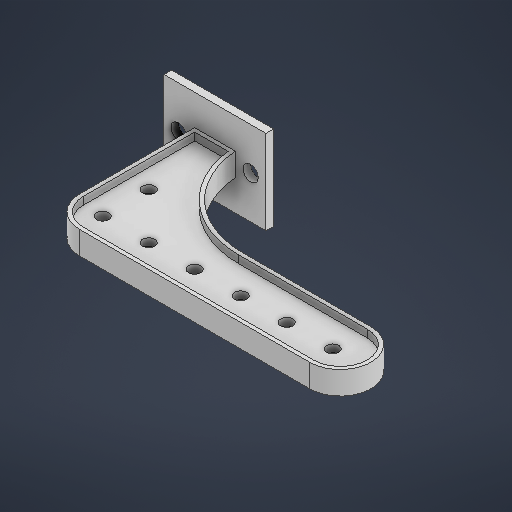
# Autodesk Inventor part: Pylon2
Saved by Autodesk Inventor 2026.1 (Build 301233000, 233)
## iProperties
Created: 2025-09-15
Part Number: Pylon2
Material: Generic
Document SubType Name: Modeling
Designer: mateo
Density: 1 g/cm^3
Appearance: Default
Author: mateo
Autodesk Inventor part; units mm, degrees
ref_plane "YZ Plane" through (0, 0, 0) normal (1, 0, 0) x (0, 1, 0)
ref_plane "XZ Plane" through (0, 0, 0) normal (0, 1, 0) x (-1, 0, 0)
ref_plane "XY Plane" through (0, 0, 0) normal (0, 0, 1) x (1, 0, 0)
sketch "Sketch1" plane through (0, 0, 0) normal (0, 1, 0) x (-1, 0, 0)
  line L0 (0, 0) -> (80, 0)
  line L1 (20, 5) -> (0, 5)
  line L2 (0, 5) -> (0, 0)
  line L3 (46.5184, 5) -> (46.5184, 80)
  circle A0 centre (26.5184, 80) radius 20
  line L4 (26.5184, 100) -> (-123.4816, 100)
  circle A1 centre (-123.4816, 80) radius 20
  line L5 (-123.4816, 60) -> (-39.7913, 60)
  arc A2 (20, 5) -> (-39.7913, 60) centre (-39.7913, 0) ccw
  line L6 (46.5184, 5) -> (66.5184, 5)
  line L7 (66.5184, 5) -> (66.5184, 0)
  line L8 (66.5184, 0) -> (46.5184, 0)
  point P0 (16.5184, 60)
  dimension "d1" = 75
  dimension "d2" = 40
  dimension "d3" = 150
  dimension "d4" = 140
  dimension "d7" = 40
  dimension "d10" = 5
  dimension "d11" = 5
  constraints: 18 end point, 6 point on circle, 4 horizontal, 3 centre point, 3 tangent, 2 parallel, 1 perpendicular, 1 point on line, 1 vertical
  measures "d1" distance of L3.start L3.end
  measures "d2" diameter of A0
  measures "d3" distance of L4.start L4.end
  measures "d4" distance of L5.start point (16.518, 60)
  measures "d7" diameter of A1
  measures "d10" distance of L6.end L7.end
  measures "d11" distance of L1.end L0.start
extrude "Extrusion1" add sketch "Sketch1" along normal blind 15
sketch "Sketch4" plane through (0, 0, 0) normal (0, -1, 0) x (1, 0, 0)
  line L0 (-26.5184, 100) -> (123.4816, 100) projected
  arc A0 (-26.5184, 100) -> (-46.5184, 80) centre (-26.5184, 80) ccw projected
  line L1 (-46.5184, 5) -> (-46.5184, 80) projected
  line L2 (-66.5184, 5) -> (-46.5184, 5) projected
  line L3 (-66.5184, 0) -> (-66.5184, 5) projected
  line L4 (0, 0) -> (-66.5184, 0) projected
  line L5 (0, 5) -> (0, 0) projected
  line L6 (-20, 5) -> (0, 5) projected
  arc A1 (39.7913, 60) -> (-20, 5) centre (39.7913, 0) ccw projected
  line L7 (123.4816, 60) -> (39.7913, 60) projected
  arc A2 (123.4816, 60) -> (123.4816, 100) centre (123.4816, 80) ccw projected
  line L8 (-20, 5) -> (-46.5184, 5)
  constraints: 2 end point, 1 horizontal
extrude "Extrusion3" add sketch "Sketch4" along normal blind 20 and the other way blind 35 contours L8 L6 L5 L4 L3 L2
sketch "Sketch5" plane through (0, 0, 0) normal (0, -1, 0) x (1, 0, 0)
  line L0 (-46.5184, 5) -> (-20, 5) projected
  arc A0 (39.7913, 60) -> (-20, 5) centre (39.7913, 0) ccw projected
  line L1 (123.4816, 60) -> (39.7913, 60) projected
  arc A1 (123.4816, 60) -> (123.4816, 100) centre (123.4816, 80) ccw projected
  line L2 (-26.5184, 100) -> (123.4816, 100) projected
  arc A2 (-26.5184, 100) -> (-46.5184, 80) centre (-26.5184, 80) ccw projected
  line L3 (-46.5184, 5) -> (-46.5184, 80) projected
  arc A3 (39.7913, 62.5) -> (-22.2571, 7.5) centre (39.7913, 0) ccw
  line L4 (-22.2571, 7.5) -> (-44.0184, 7.5)
  line L5 (-44.0184, 7.5) -> (-44.0184, 80)
  arc A4 (-26.5184, 97.5) -> (-44.0184, 80) centre (-26.5184, 80) ccw
  line L6 (-26.5184, 97.5) -> (123.4816, 97.5)
  arc A5 (123.4816, 62.5) -> (123.4816, 97.5) centre (123.4816, 80) ccw
  line L7 (123.4816, 62.5) -> (39.7913, 62.5)
  point P0 (0, 0)
  dimension "d29" = 2.5
  constraints: 8 end point, 6 point on circle, 3 centre point, 6 other
  measures "d29" distance between parallel lines of L1 L7
extrude "Extrusion4" cut sketch "Sketch5" against normal blind 5 contours A3 L4 L5 A4 L6 A5 L7
sketch "Sketch6" plane through (0, 15, 0) normal (0, 1, 0) x (1, 0, 0)
  line L0 (-20, -5) -> (-46.5184, -5) projected
  line L1 (-46.5184, -5) -> (-46.5184, -80) projected
  arc A0 (-46.5184, -80) -> (-26.5184, -100) centre (-26.5184, -80) ccw projected
  line L2 (-26.5184, -100) -> (123.4816, -100) projected
  arc A1 (123.4816, -100) -> (123.4816, -60) centre (123.4816, -80) ccw projected
  line L3 (123.4816, -60) -> (39.7913, -60) projected
  arc A2 (-20, -5) -> (39.7913, -60) centre (39.7913, 0) ccw projected
  line L4 (-44.0184, -80) -> (-44.0184, -7.5)
  line L5 (-44.0184, -7.5) -> (-22.2571, -7.5)
  arc A3 (-22.2571, -7.5) -> (39.7913, -62.5) centre (39.7913, 0) ccw
  line L6 (39.7913, -62.5) -> (123.4816, -62.5)
  arc A4 (123.4816, -97.5) -> (123.4816, -62.5) centre (123.4816, -80) ccw
  line L7 (123.4816, -97.5) -> (-26.5184, -97.5)
  arc A5 (-44.0184, -80) -> (-26.5184, -97.5) centre (-26.5184, -80) ccw
  point P0 (0, 0)
  dimension "d32" = 2.5
  constraints: 8 end point, 6 point on circle, 3 centre point, 6 other
  measures "d32" distance between parallel lines of L1 L4
extrude "Extrusion5" cut sketch "Sketch6" against normal blind 5 contours L4 L5 A3 L6 A4 L7 A5
sketch "Sketch7" plane through (0, 10, 0) normal (0, 1, 0) x (1, 0, 0)
  line L0 (123.4816, -97.5) -> (-26.5184, -97.5) projected
  line L1 (39.7913, -62.5) -> (123.4816, -62.5) projected
  line L2 (123.4816, -62.5) -> (39.7913, -62.5) projected
  line L3 (118.4816, -62.5) -> (118.4816, -80)
  circle A0 centre (118.4816, -80) radius 4
  line L4 (-44.0184, -80) -> (-44.0184, -7.5) projected
  circle A1 centre (88.4816, -80) radius 4
  circle A2 centre (58.4816, -80) radius 4
  circle A3 centre (28.4816, -80) radius 4
  circle A4 centre (-1.5184, -80) radius 4
  circle A5 centre (-31.5184, -80) radius 4
  arc A6 (123.4816, -97.5) -> (123.4816, -62.5) centre (123.4816, -80) ccw projected
  circle A7 centre (-31.5184, -50) radius 4
  point P0 (0, 0)
  dimension "d35" = 35
  dimension "d36" = 17.5
  dimension "d37" = 8
  dimension "d39" = 8
  dimension "d41" = 8
  dimension "d43" = 8
  dimension "d45" = 8
  dimension "d46" = 8
  dimension "d47" = 30
  dimension "d48" = 30
  dimension "d49" = 30
  dimension "d50" = 30
  dimension "d51" = 5
  dimension "d52" = 30
  dimension "d53" = 8
  dimension "d54" = 30
  constraints: 7 centre point, 2 end point, 1 coincident, 1 perpendicular, 1 point on line
  measures "d35" distance between parallel lines of L0 L1
  measures "d36" distance of L3.start L3.end
  measures "d37" diameter of A0
  measures "d39" diameter of A1
  measures "d41" diameter of A2
  measures "d43" diameter of A3
  measures "d45" diameter of A4
  measures "d46" diameter of A5
  measures "d47" distance of A3.centre A4.centre
  measures "d48" distance of A4.centre A5.centre
  measures "d49" distance of A3.centre A2.centre
  measures "d50" distance of A2.centre A1.centre
  measures "d51" distance of A6.centre A0.centre
  measures "d52" distance of A1.centre A0.centre
  measures "d53" diameter of A7
  measures "d54" distance of A5.centre A7.centre
extrude "Extrusion6" cut sketch "Sketch7" against normal blind 8
sketch "Sketch8" plane through (0, 35, 0) normal (0, 0, -1) x (-1, 0, 0)
  line L0 (20, -20) -> (46.5184, -20) projected
  line L1 (46.5184, -35) -> (20, -35) projected
  line L2 (20, -35) -> (20, -20) projected
  line L3 (46.5184, -35) -> (46.5184, -20) projected
  line L4 (0, 0) -> (66.5184, 0) projected
  line L5 (66.5184, -55) -> (0, -55) projected
  circle A0 centre (10, -27.5) radius 5
  circle A1 centre (57.0363, -27.5) radius 5
  point P0 (0, -35)
  dimension "d57" = 20
  dimension "d58" = 20
  dimension "d59" = 10
  dimension "d60" = 10
  dimension "d61" = 10
  constraints: 2 centre point
  measures "d57" distance between parallel lines of L4 L0
  measures "d58" distance between parallel lines of L5 L1
  measures "d59" diameter of A0
  measures "d60" diameter of A1
  measures "d61" distance from line of L2 A0.centre
extrude "Extrusion7" cut sketch "Sketch8" against normal blind 10 contours A0 | A1
equation "\"d55\" = d39"
body "Solid1"
